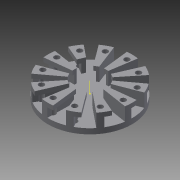
# Autodesk Inventor part: male bayonet connector 12
Saved by Autodesk Inventor 2015 (Build 190159000, 159)
## iProperties
Created: 2014-06-11
Part Number: male bayonet connector 12
Material: Generic
Document SubType Name: Modeling
Designer: ericd_000
Density: 1 g/cm^3
Appearance: Default
Author: ericd_000
Autodesk Inventor part; units mm, degrees
ref_plane "YZ Plane" through (0, 0, 0) normal (1, 0, 0) x (0, 1, 0)
ref_plane "XZ Plane" through (0, 0, 0) normal (0, 1, 0) x (-1, 0, 0)
ref_plane "XY Plane" through (0, 0, 0) normal (0, 0, 1) x (1, 0, 0)
sketch "Sketch19" plane through (0, 0, 0) normal (0, 0, 1) x (1, 0, 0)
  circle A0 centre (0, 0) radius 39.5
  dimension "d94" = 79
  constraints: 1 centre point, 1 coincident
  measures "d94" diameter of A0
extrude "Extrusion20" add sketch "Sketch19" along normal blind 5
sketch "Sketch21" plane through (0, 0, 5) normal (0, 0, 1) x (1, 0, 0)
  point P0 (0, 0)
sketch "Sketch23" plane through (0, 0, 5) normal (0, 0, 1) x (1, 0, 0)
  line L0 (0, 0) -> (20.2843, 33.8939) construction
  circle A0 centre (0, 0) radius 39.5 construction
  line L1 (0, 0) -> (24.804, 30.7411) construction
  circle A1 centre (0, 0) radius 39.5 construction
  line L2 (24.804, 30.7411) -> (9.4735, 11.7411)
  line L3 (9.4735, 11.7411) -> (7.6719, 12.8193)
  line L4 (7.6719, 12.8193) -> (20.2843, 33.8939)
  arc A2 (24.804, 30.7411) -> (20.2843, 33.8939) centre (0, 0) ccw
  dimension "d105" = 172
  dimension "d106" = 19
  constraints: 10 end point, 2 collinear, 2 point on circle, 1 centre point, 1 perpendicular, 5 other
  measures "d105" angle of L0 L1
  measures "d106" vertical distance of L1.end L2.end
extrude "Extrusion21" add sketch "Sketch23" along normal blind 12.5
sketch "Sketch26" plane through (7.6719, 12.8193, 5) normal (-0.8580744, 0.5135254, 0) x (0, 0, 1)
  line L0 (12.5, 24.5604) -> (12.5, 0)
  line L1 (12.5, 24.5604) -> (8.5, 24.5604)
  line L2 (0, 24.5604) -> (12.5, 24.5604) projected
  line L3 (0, 0) -> (12.5, 0) projected
  line L4 (8.5, 0) -> (12.5, 0)
  line L5 (8.5, 24.5604) -> (8.5, 0)
  line L6 (-8.5, -14.9396) -> (16, -14.9396) projected
  point P0 (-5, -14.9396)
  dimension "d122" = 4
  dimension "d123" = 4
  constraints: 8 end point, 2 point on line, 1 collinear, 1 vertical
  measures "d122" distance of L0.start L1.end
  measures "d123" distance of L4.start L0.end
revolve "Revolution2" add sketch "Sketch26" angle 7.5 about axis through (0, 0, 5) along (0, 0, 1)
sketch "Sketch25" plane through (0, 0, 17.5) normal (0, 0, 1) x (1, 0, 0)
  circle A0 centre (17.9697, 27.6783) radius 2.5
  line L0 (17.9697, 27.6783) -> (0, 0) construction
  line L1 (5.933, 13.711) -> (15.6867, 36.2516) projected
  dimension "d112" = 5
  dimension "d116" = 33
  dimension "d125" = 5.5
  constraints: 2 end point, 1 centre point
  measures "d112" diameter of A0
  measures "d116" distance of L0.start L0.end
  measures "d125" distance from line of L0.start L1
extrude "Extrusion22" cut sketch "Sketch25" against normal through all
sketch "Sketch27" plane through (0, 0, 17.5) normal (0, 0, 1) x (1, 0, 0)
  line L0 (7.6719, 12.8193) -> (9.4735, 11.7411) projected
  line L1 (7.6719, 12.8193) -> (5.933, 13.711)
  line L2 (5.933, 13.711) -> (19.7656, 45.678)
  line L3 (5.933, 13.711) -> (15.6867, 36.2516) projected
  line L4 (19.7656, 45.678) -> (7.5595, 12.8769)
  point P0 (0, 0)
  constraints: 7 end point, 2 point on line
extrude "Extrusion23" [suppressed]
pattern_circular "Circular Pattern2" count 12 over 360 about axis through (0, 0, 5) along (0, 0, 1) of "Extrusion21", "Revolution2", "Extrusion22"
sketch "Sketch29" plane through (0, 0, 5) normal (0, 0, 1) x (1, 0, 0)
  circle A0 centre (0, 0) radius 59
  line L0 (0, 0) -> (-30.7411, 24.804)
  line L1 (0, 0) -> (-33.8939, 20.2843)
  line L2 (-12.8193, 7.6719) -> (-33.8939, 20.2843) projected
  arc A1 (-34.5136, -19.2109) -> (-24.804, -30.7411) centre (0, 0) ccw projected
  point P0 (-30.1767, 18.0596)
  dimension "d135" = 118
  constraints: 4 end point, 1 centre point, 1 coincident, 1 collinear, 1 concentric
  measures "d135" diameter of A0
extrude "Extrusion26" [suppressed]
sketch "Sketch30" plane through (0, 0, 5) normal (0, 0, -1) x (-1, 0, 0)
  line L0 (-109.7485, 105.489) -> (97.8298, 105.489)
  line L1 (97.8298, 105.489) -> (97.8298, -69.3705)
  line L2 (97.8298, -69.3705) -> (-109.7485, -69.3705)
  line L3 (-109.7485, -69.3705) -> (-109.7485, 105.489)
  line L4 (32.0383, -2.0031) -> (28.8173, 14.5454)
  line L5 (28.8173, 14.5454) -> (71.7406, 33.7946)
  line L6 (71.7406, 33.7946) -> (71.7406, -3.6949)
  line L7 (71.7406, -3.6949) -> (32.0383, -2.0031)
  point P0 (0, 0)
  constraints: 16 end point, 2 parallel, 1 horizontal, 1 perpendicular, 1 vertical
extrude "Extrusion27" [suppressed]
sketch "Sketch31" plane through (-36.2516, 15.6867, 17.5) normal (0, 0, 1) x (0.917762, -0.3971309, 0)
  line L0 (16, 0) -> (20, 0)
  line L1 (20, 0) -> (20, 3)
  line L2 (20, 3) -> (16, 3)
  line L3 (16, 3) -> (16, 0)
  line L4 (24.5604, 0) -> (0, 0) projected
  point P0 (39.5, 0)
  point P1 (24.7502, 0)
  dimension "d148" = 16
  dimension "d149" = 4
  dimension "d150" = 3
  constraints: 8 end point, 2 parallel, 1 collinear, 1 horizontal, 1 perpendicular
  measures "d148" distance from line of L3 L4.end
  measures "d149" distance of L1.end L2.end
  measures "d150" distance of L0.end L1.end
extrude "Extrusion28" cut sketch "Sketch31" against normal up to surface (4 mm away)
sketch "Sketch32" plane through (-30.7411, 24.804, 17.5) normal (0, 0, 1) x (0.7782548, -0.6279487, 0)
  line L0 (16.8547, -6.2801) -> (15.1131, 0)
  line L1 (0, 0) -> (24.4136, 0) projected
  line L2 (16.8547, -6.2801) -> (16.053, -3.3892) projected
  line L3 (16.8547, -6.2801) -> (25.1038, -3.9924)
  line L4 (25.1038, -3.9924) -> (24.4136, 0)
  line L5 (15.1131, 0) -> (24.4136, 0)
  line L6 (16.8547, -6.2801) -> (16.5656, -6.3603)
  line L7 (16.8547, -6.2801) -> (1.4366, -10.5559) projected
  line L8 (14.8017, 0) -> (15.1131, 0)
  line L9 (15.1131, 0) -> (14.8017, 0)
  line L10 (16.5656, -6.3603) -> (14.8017, 0)
  point P0 (39.5, 0)
  dimension "d153" = 0.3
  constraints: 16 end point, 4 collinear, 3 point on line, 1 parallel
  measures "d153" distance between parallel lines of L10 L0
extrude "Extrusion30" cut sketch "Sketch32" against normal up to surface (12.5 mm away)
body "Solid2"
